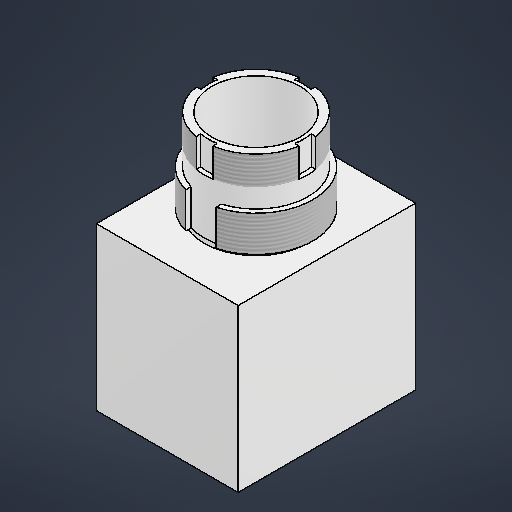
# Autodesk Inventor part: Body
Saved by Autodesk Inventor 2026 (Build 300175050, 175E)
## iProperties
Created: 2025-06-28
Part Number: Body
Material: ABS Plastic
Document SubType Name: Modeling
Designer: Joshua Eah
Density: 1.06 g/cm^3
Appearance: Smooth - White
Author: Joshua Eah
Autodesk Inventor part; units mm, degrees
ref_plane "YZ Plane" through (0, 0, 0) normal (1, 0, 0) x (0, 1, 0)
ref_plane "XZ Plane" through (0, 0, 0) normal (0, 1, 0) x (-1, 0, 0)
ref_plane "XY Plane" through (0, 0, 0) normal (0, 0, 1) x (1, 0, 0)
sketch "Sketch1" plane through (0, 0, 0) normal (0, 1, 0) x (-1, 0, 0)
  line L0 (0, 0) -> (-29.7815, 0)
  line L1 (-29.7815, 0) -> (-29.7815, -37.2745)
  line L2 (-29.7815, -37.2745) -> (0, -37.2745)
  line L3 (0, -37.2745) -> (0, 0)
  line L4 (-14.8907, -37.2745) -> (-14.8907, 0)
  line L5 (0, -18.6373) -> (-29.7815, -18.6373)
  circle A0 centre (-14.8907, -18.6373) radius 10.8903
  dimension "d0" = 29.7815
  dimension "d1" = 37.2745
  dimension "d2" = 21.7805
  constraints: 12 end point, 5 midpoint, 2 parallel, 1 centre point, 1 horizontal, 1 perpendicular
  measures "d0" distance of L2.end L1.end
  measures "d1" distance of L1.end L0.end
  measures "d2" diameter of A0
extrude "Extrusion1" add sketch "Sketch1" against normal blind 34
extrude "Extrusion2" add sketch "Sketch1" along normal blind 1 contours A0 L5 L4 | L4 L5 A0 | A0 L4 L5 | L4 A0 L5
sketch "Sketch2" plane through (14.8907, 1, -18.6373) normal (0, 1, 0) x (1, 0, 0)
  circle A0 centre (0, 0) radius 12
  dimension "d9" = 24
  constraints: 1 centre point
  measures "d9" diameter of A0
extrude "Extrusion3" add sketch "Sketch2" along normal blind 7.5
sketch "Sketch3" plane through (14.8907, 8.5, -18.6373) normal (0, 1, 0) x (1, 0, 0)
  circle A0 centre (0, 0) radius 10.925
  circle A1 centre (0, 0) radius 12 projected
  line L0 (-3.175, -12) -> (3.175, -12)
  line L1 (3.175, -12) -> (3.175, 12)
  line L2 (3.175, 12) -> (-3.175, 12)
  line L3 (-3.175, 12) -> (-3.175, -12)
  line L4 (-3.175, -12) -> (3.175, 12) construction
  line L5 (3.175, -12) -> (-3.175, 12) construction
  point P0 (-3.175, -11.5724)
  point P1 (3.175, -11.5724)
  point P2 (-3.175, 11.5724)
  point P3 (3.175, 11.5724)
  point P4 (0, -12)
  point P5 (0, 12)
  point P6 (-3.175, -10.4535)
  point P7 (3.175, -10.4535)
  dimension "d12" = 21.85
  dimension "d21" = 6.35
  constraints: 12 end point, 2 midpoint, 2 parallel, 1 centre point, 1 concentric, 1 horizontal, 1 perpendicular, 1 tangent
  measures "d12" diameter of A0
  measures "d21" distance of L2.end L1.end
extrude "Extrusion4" add sketch "Sketch3" along normal blind 10 contours A0 L1 | L1 A0 L3 | L3 A0
thread "Thread2" size "M24x0.75" class "6g" standard "ANSI Metric M Profile" full length
thread "Thread3" size "M22x0.75" class "6g" standard "ANSI Metric M Profile" length 10.0076 offset 4
extrude "Extrusion5" cut sketch "Sketch3" against normal up to surface (7.5 mm away) contours L1 A1 L3 A0 picked at (0, -11.2482)
sketch "Sketch4" plane through (14.8907, 18.5, -18.6373) normal (0, 1, 0) x (1, 0, 0)
  circle A0 centre (0, 0) radius 10.925 projected
  line L0 (-1.75, 10.925) -> (1.75, 10.925)
  line L1 (1.75, 10.925) -> (1.75, -10.925)
  line L2 (1.75, -10.925) -> (-1.75, -10.925)
  line L3 (-1.75, -10.925) -> (-1.75, 10.925)
  line L4 (-1.75, 10.925) -> (1.75, -10.925) construction
  line L5 (1.75, 10.925) -> (-1.75, -10.925) construction
  circle A1 centre (0, 0) radius 10
  line L6 (-10.925, -1.75) -> (10.925, -1.75)
  line L7 (10.925, -1.75) -> (10.925, 1.75)
  line L8 (10.925, 1.75) -> (-10.925, 1.75)
  line L9 (-10.925, 1.75) -> (-10.925, -1.75)
  line L10 (-10.925, -1.75) -> (10.925, 1.75) construction
  line L11 (10.925, -1.75) -> (-10.925, 1.75) construction
  point P0 (-9.8457, 1.75)
  point P1 (-10.7839, 1.75)
  point P2 (-10.7839, -1.75)
  point P3 (-9.8457, -1.75)
  point P4 (-1.75, 9.8457)
  point P5 (1.75, 9.8457)
  point P6 (1.75, 10.7839)
  point P7 (-1.75, 10.7839)
  point P8 (10.7839, 1.75)
  point P9 (9.8457, 1.75)
  point P10 (9.8457, -1.75)
  point P11 (10.7839, -1.75)
  point P12 (1.75, -9.8457)
  point P13 (-1.75, -9.8457)
  point P14 (-1.75, -10.7839)
  point P15 (1.75, -10.7839)
  dimension "d25" = 3.5
  dimension "d26" = 20
  dimension "d27" = 3.5
  constraints: 24 end point, 4 midpoint, 4 parallel, 2 horizontal, 2 perpendicular, 2 tangent, 1 centre point, 1 coincident
  measures "d25" distance of L1.end L2.end
  measures "d26" diameter of A1
  measures "d27" distance of L7.end L6.end
extrude "Extrusion6" cut sketch "Sketch4" against normal blind 6 contours A0 L6 A1 L8 | L1 A1 L3 A0 | A0 L3 A1 L1 | L8 A1 L6 A0
hole "Hole1" at (14.8907, 18.5, -18.6373) direction (0, -1, 0) diameter 18.5 depth 18.5
body "Solid1"
